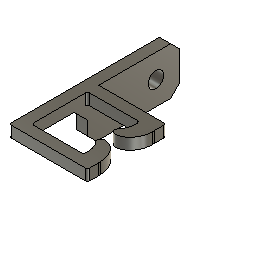
vertical (Autodesk Fusion 360 design; units mm, degrees)
Autodesk Fusion 360 part; units mm, degrees
sketch "rail-profile" plane through (0, 0, 0) normal (0, 1, 0) x (1, 0, 0)
  line L0 (-13.3, -34.5) -> (-13.3, -17.775)
  line L1 (-11.8, -16.275) -> (-1.5, -16.275)
  line L2 (0, -14.775) -> (0, 0)
  line L3 (0, 0) -> (5, 0) construction
  arc A0 (-11.8, -16.275) -> (-13.3, -17.775) centre (-11.8, -17.775) ccw
  arc A1 (-1.5, -16.275) -> (0, -14.775) centre (-1.5, -14.775) ccw
  line L4 (-12, -34.5) -> (-12, -17.775)
  arc A2 (-11.8, -17.575) -> (-12, -17.775) centre (-11.8, -17.775) ccw
  line L5 (-11.8, -17.575) -> (-1.5, -17.575)
  arc A3 (-1.5, -17.575) -> (1.3, -14.775) centre (-1.5, -14.775) ccw
  line L6 (1.3, -14.775) -> (1.3, 0)
  line L7 (-13.3, -34.5) -> (-12, -34.5)
  line L8 (0, 14.775) -> (0, 0)
  arc A4 (0, 14.775) -> (-1.5, 16.275) centre (-1.5, 14.775) ccw
  line L9 (-11.8, 16.275) -> (-1.5, 16.275)
  arc A5 (-13.3, 17.775) -> (-11.8, 16.275) centre (-11.8, 17.775) ccw
  line L10 (-13.3, 34.5) -> (-13.3, 17.775)
  line L11 (-13.3, 34.5) -> (-12, 34.5)
  line L12 (-12, 34.5) -> (-12, 17.775)
  arc A6 (-12, 17.775) -> (-11.8, 17.575) centre (-11.8, 17.775) ccw
  line L13 (-11.8, 17.575) -> (-1.5, 17.575)
  arc A7 (1.3, 14.775) -> (-1.5, 17.575) centre (-1.5, 14.775) ccw
  line L14 (1.3, 14.775) -> (1.3, 0)
  point P0 (-13.3, -16.275)
  point P1 (0, -16.275)
  dimension "d4" = 16.275
  dimension "d5" = 13.3
  dimension "d7" = 34.5
  dimension "d8" = 1.5
  dimension "d9" = 1.5
  dimension "d10" = 1.3
  constraint vertical L0
  constraint perpendicular L0 L1
  constraint perpendicular L1 L2
  constraint coincident L2.end L3.start
  constraint perpendicular L2 L3
  constraint coincident P0 L0
  constraint coincident P0 L1
  constraint tangent L0 A0
  constraint tangent L1 A0
  constraint coincident P1 L1
  constraint coincident P1 L2
  constraint tangent L1 A1
  constraint tangent L2 A1
  constraint symmetric L0.start L3 L10.start
  constraint symmetric L2.end L3 L8.end
  constraint symmetric L3 L0.end A5.start
  constraint symmetric L3 L1.start L9.start
  constraint symmetric L3 A0 A5
  constraint symmetric L3 L1.end A4.end
  constraint symmetric L3 L2.start L8.start
  constraint symmetric L3 A1 A4
  constraint symmetric L3 L4.start L11.end
  constraint symmetric L3 L4.end L12.end
  constraint symmetric L3 A2.start A6.end
  constraint symmetric L3 A2 A6
  constraint symmetric L3 L5.end L13.end
  constraint symmetric L3 A3.end A7.start
  constraint symmetric L3 A3 A7
  constraint symmetric L3 L6.end L14.end
  measures "d4" distance of L1 L3
  measures "d5" distance of P0 P1
  measures "d7" vertical distance of L0.start L3.end
  measures "d8" radius of A0
  measures "d9" radius of A1
extrude "Extrude1" add sketch "rail-profile" along normal blind 60 makes body 1
sketch "cutoout-profile" plane through (0, 0, 0) normal (-1, 0, 0) x (0, -1, 0)
  line L0 (0, -14.775) -> (0, 14.775)
  line L1 (0, 14.775) -> (-60, 14.775)
  line L2 (-60, 14.775) -> (-60, -14.775)
  line L3 (-60, -14.775) -> (0, -14.775)
  line L4 (-50.85, 4.575) -> (-60, 4.575)
  line L5 (-60, 4.575) -> (-60, -4.575)
  line L6 (-60, -4.575) -> (-50.85, -4.575)
  line L7 (-50.85, -4.575) -> (-50.85, 4.575)
  line L8 (-50.85, 4.575) -> (-60, -4.575) construction
  line L9 (-60, 4.575) -> (-50.85, -4.575) construction
  line L10 (-60, 0) -> (0, 0) construction
  line L11 (-40, -4.575) -> (-30.85, -4.575)
  line L12 (-30.85, -4.575) -> (-30.85, 4.575)
  line L13 (-30.85, 4.575) -> (-40, 4.575)
  line L14 (-40, 4.575) -> (-40, -4.575)
  line L15 (-20, -4.575) -> (-10.85, -4.575)
  line L16 (-10.85, -4.575) -> (-10.85, 4.575)
  line L17 (-10.85, 4.575) -> (-20, 4.575)
  line L18 (-20, 4.575) -> (-20, -4.575)
  point P0 (-55.425, 0)
  dimension "d13" = 9.15
  dimension "d14" = 9.15
  dimension "d24" = 60
  dimension "d25" = 0
  constraint horizontal L4
  constraint perpendicular L4 L5
  constraint parallel L4 L6
  constraint parallel L5 L7
  constraint coincident L8 P0
  constraint coincident L9 P0
  constraint midpoint L2 L10.start
  constraint coincident L10.end origin
  constraint coincident P0 L10
  constraint coincident L5 L10.start
  measures "d13" distance of L5.end L6.end
  measures "d14" distance of L4.end L5.end
extrude "Extrude2" cut sketch "cutoout-profile" against normal up to surface (1.3 mm away) contours L2 L4 L5 L6 L7 | L11 L12 L13 L14 | L15 L16 L17 L18 bodies 1
sketch "rail-body" plane through (1.3, 0, 0) normal (1, 0, 0) x (0, 1, 0) in component "cable-component"
  line L0 (50.85, 4.575) -> (60, 4.575)
  line L1 (60, 4.575) -> (60, 14.775)
  line L2 (60, 14.775) -> (0, 14.775)
  line L3 (0, 14.775) -> (0, -14.775)
  line L4 (0, -14.775) -> (60, -14.775)
  line L5 (60, -14.775) -> (60, -4.575)
  line L6 (60, -4.575) -> (50.85, -4.575)
  line L7 (50.85, -4.575) -> (50.85, 4.575)
  line L8 (30.85, 4.575) -> (40, 4.575)
  line L9 (40, 4.575) -> (40, -4.575)
  line L10 (40, -4.575) -> (30.85, -4.575)
  line L11 (30.85, -4.575) -> (30.85, 4.575)
  line L12 (10.85, 4.575) -> (20, 4.575)
  line L13 (20, 4.575) -> (20, -4.575)
  line L14 (20, -4.575) -> (10.85, -4.575)
  line L15 (10.85, -4.575) -> (10.85, 4.575)
  circle A0 centre (15.425, 0) radius 3.5
  line L16 (10.85, 4.575) -> (20, -4.575) construction
  line L17 (20, 4.575) -> (10.85, -4.575) construction
  line L18 (30.85, 4.575) -> (40, -4.575) construction
  line L19 (40, 4.575) -> (30.85, -4.575) construction
  circle A1 centre (35.425, 0) radius 3.5
  line L20 (4.85, 10.575) -> (46, 10.575)
  line L21 (46, 10.575) -> (46, -10.575)
  line L22 (46, -10.575) -> (4.85, -10.575)
  line L23 (4.85, -10.575) -> (4.85, 10.575)
  point P0 (15.425, 0)
  point P1 (35.425, 0)
  dimension "d28" = 7
  dimension "d30" = 7
  dimension "d31" = 6
  dimension "d32" = 6
  dimension "d33" = 6
  dimension "d34" = 6
  constraint coincident L12.start L15.end
  constraint coincident L13.end L14.start
  constraint coincident L12.end L13.start
  constraint coincident L14.end L15.start
  constraint midpoint L16 P0
  constraint coincident P0 A0.centre
  constraint coincident L8.start L11.end
  constraint coincident L9.end L10.start
  constraint coincident L8.end L9.start
  constraint coincident L10.end L11.start
  constraint midpoint L18 P1
  constraint coincident P1 A1.centre
  constraint horizontal L20
  constraint vertical L21
  constraint horizontal L22
  constraint vertical L23
  measures "d28" diameter of A0
  measures "d30" diameter of A1
  measures "d31" distance of L15 L23
  measures "d32" distance of L9 L21
  measures "d33" distance of L14 L22
  measures "d34" distance of L12 L20
extrude "Extrude1'" add sketch "rail-body" along normal blind 5 separate body contours L8 L9 L10 L11 | L12 L13 L14 L15 | L20 L21 L22 L23 makes body 2 in component "cable-component"
sketch "hook-body" plane through (0, 0, 10.575) normal (0, 0, 1) x (-1, 0, 0) in component "cable-component"
  line L0 (-1.3, -46) -> (-1.3, -4.85)
  line L1 (-1.3, -4.85) -> (-6.3, -4.85)
  line L2 (-6.3, -4.85) -> (-6.3, -46)
  line L3 (-6.3, -46) -> (-1.3, -46)
  line L4 (-6.3, -18.925) -> (-6.3, -11.925)
  line L5 (-6.3, -38.925) -> (-6.3, -31.925)
  line L6 (-1.3, -4.85) -> (-1.3, 25.15)
  line L7 (-1.3, 25.15) -> (-36.3, 25.15)
  line L8 (-36.3, 25.15) -> (-36.3, 20.15)
  line L9 (-36.3, 20.15) -> (-6.3, 20.15)
  line L10 (-1.3, -9.85) -> (-36.3, -9.85)
  line L11 (-1.3, -4.85) -> (-36.2454, -4.85)
  line L12 (-6.3, 20.15) -> (-6.3, -4.85)
  line L13 (-1.3, -4.85) -> (-1.3, -9.85)
  line L14 (-36.2454, -4.85) -> (-36.3, -9.85)
  dimension "d73" = 35
  dimension "d82" = 5
  dimension "d84" = 5
  dimension "d86" = 35
  constraint coincident L0.end L1.start
  constraint perpendicular L1 L6
  constraint perpendicular L6 L7
  constraint perpendicular L7 L8
  constraint coincident L0 L10.start
  constraint perpendicular L0 L10
  constraint horizontal L11
  constraint coincident L1.end L2.start
  constraint perpendicular L1 L12
  measures "d73" distance of L6 L8
  measures "d82" distance of L7 L9
  measures "d84" distance of L10 L11
  measures "d86" distance of L7 L10
extrude "Extrude3" add sketch "hook-body" against normal blind 5 contours L1 L6 L7 L8 L9 L11 L12 | L2 L10 L11 L14 bodies 2 in component "cable-component"
sketch "hook-profile" plane through (0, 0, 10.575) normal (0, 0, 1) x (-1, 0, 0) in component "cable-component"
  line L0 (-1.3, -46) -> (-1.3, 25.15)
  line L1 (-1.3, 25.15) -> (-36.3, 25.15)
  line L2 (-36.3, 25.15) -> (-36.3, 20.15)
  line L3 (-36.3, 20.15) -> (-6.3, 20.15)
  line L4 (-36.3, -9.85) -> (-6.3, -9.85)
  line L5 (-6.3, -9.85) -> (-6.3, -46)
  line L6 (-6.3, -46) -> (-1.3, -46)
  line L7 (-29.51, -3.85) -> (-36.2454, -3.85)
  spline S0 degree 5 poles (-36.2454, -3.85) (-36.2422, -3.7398) (-36.2342, -3.519) (-36.2171, -3.1868) (-36.1838, -2.7425) (-36.1211, -2.1886) (-36.0333, -1.6413) (-35.9167, -1.1062) (-35.7694, -0.588) (-35.5924, -0.09) (-35.3903, 0.3872) (-35.1691, 0.8444) (-34.935, 1.2835) (-34.692, 1.7065) (-34.4408, 2.1153) (-34.1762, 2.5107) (-33.8891, 2.8926) (-33.5692, 3.2598) (-33.2076, 3.6106) (-32.7989, 3.9423) (-32.3446, 4.252) (-31.8525, 4.536) (-31.3346, 4.7901) (-30.8054, 5.0093) (-30.2798, 5.188) (-29.7712, 5.3193) (-29.2893, 5.3956) (-28.8411, 5.4092) (-28.4314, 5.3544) (-28.0646, 5.2289) (-27.7456, 5.0354) (-27.4806, 4.7835) (-27.2769, 4.4876) (-27.1409, 4.1648) (-27.0781, 3.8331) (-27.0911, 3.5096) (-27.1789, 3.2064) (-27.3352, 2.9276) (-27.5468, 2.665) (-27.7932, 2.3973) (-28.0525, 2.1) (-28.3047, 1.7523) (-28.5366, 1.3455) (-28.7453, 0.8894) (-28.9331, 0.4032) (-29.1035, -0.0933) (-29.2575, -0.586) (-29.3866, -1.0791) (-29.4756, -1.5936) (-29.5254, -2.1319) (-29.5418, -2.6919) (-29.5361, -3.1515) (-29.5251, -3.4998) (-29.5154, -3.7331) (-29.51, -3.85) knots 0 0 0 0 0 0 0.02 0.04 0.06 0.08 0.1 0.12 0.14 0.16 0.18 0.2 0.22 0.24 0.26 0.28 0.3 0.32 0.34 0.36 0.38 0.4 0.42 0.44 0.46 0.48 0.5 0.52 0.54 0.56 0.58 0.6 0.62 0.64 0.66 0.68 0.7 0.72 0.74 0.76 0.78 0.8 0.82 0.84 0.86 0.88 0.9 0.92 0.94 0.96 0.98 1 1 1 1 1 1
  line L8 (-36.3068, -5.9745) -> (-36.184, -1.7255)
  line L9 (-28.7421, 1.2922) -> (-29.8225, -2.6884)
  line L10 (-29.6154, -1.588) -> (-29.4045, -6.112)
  line L11 (-6.3, 20.15) -> (-6.3, -4.85)
  line L12 (-6.3, -4.85) -> (-36.2454, -4.85)
  line L13 (-36.2454, -4.85) -> (-36.3, -9.85)
  line L14 (-36.2454, -4.85) -> (-36.2454, -3.85)
  line L15 (-6.3, 7.65) -> (-36.3271, 7.6919) construction
  line L16 (-29.51, -3.85) -> (-29.51, -4.85)
  spline S1 degree 5 poles (-36.2132, 19.2335) (-36.2103, 19.1233) (-36.2029, 18.9025) (-36.1868, 18.5703) (-36.1547, 18.1258) (-36.0936, 17.5717) (-36.0072, 17.0242) (-35.8922, 16.4888) (-35.7463, 15.9702) (-35.5707, 15.4717) (-35.3699, 14.9939) (-35.15, 14.5361) (-34.9171, 14.0964) (-34.6753, 13.6727) (-34.4253, 13.2632) (-34.1618, 12.867) (-33.8758, 12.4843) (-33.5569, 12.1162) (-33.1962, 11.7645) (-32.7885, 11.4316) (-32.335, 11.1207) (-31.8437, 10.8353) (-31.3265, 10.5798) (-30.798, 10.359) (-30.2729, 10.1789) (-29.7646, 10.0462) (-29.2829, 9.9685) (-28.8347, 9.9537) (-28.4249, 10.0073) (-28.0578, 10.1318) (-27.7382, 10.3244) (-27.4726, 10.5755) (-27.268, 10.8709) (-27.1311, 11.1933) (-27.0673, 11.5248) (-27.0794, 11.8484) (-27.1664, 12.1519) (-27.322, 12.431) (-27.5328, 12.6942) (-27.7785, 12.9626) (-28.0369, 13.2606) (-28.2882, 13.6091) (-28.519, 14.0165) (-28.7263, 14.4732) (-28.9128, 14.9599) (-29.0818, 15.4569) (-29.2344, 15.95) (-29.3622, 16.4434) (-29.4497, 16.9582) (-29.4981, 17.4966) (-29.5129, 18.0567) (-29.5059, 18.5163) (-29.4939, 18.8646) (-29.4836, 19.0978) (-29.4778, 19.2147) knots 0 0 0 0 0 0 0.02 0.04 0.06 0.08 0.1 0.12 0.14 0.16 0.18 0.2 0.22 0.24 0.26 0.28 0.3 0.32 0.34 0.36 0.38 0.4 0.42 0.44 0.46 0.48 0.5 0.52 0.54 0.56 0.58 0.6 0.62 0.64 0.66 0.68 0.7 0.72 0.74 0.76 0.78 0.8 0.82 0.84 0.86 0.88 0.9 0.92 0.94 0.96 0.98 1 1 1 1 1 1
  line L17 (-36.2687, 21.3582) -> (-36.1577, 17.1088)
  line L18 (-28.7243, 14.0703) -> (-29.7936, 18.054)
  line L19 (-29.5896, 16.953) -> (-29.366, 21.4764)
  line L20 (-29.4778, 19.2147) -> (-29.475, 20.2147)
  line L21 (-36.2104, 20.2335) -> (-36.2132, 19.2335)
  point P0 (-36.3271, 7.6919)
  point P1 (-27.2909, 3.0236)
  point P2 (-34.6419, 1.7831)
  point P3 (-28.2703, 1.7831)
  point P4 (-33.0367, 3.7418)
  point P5 (-35.7948, -0.6981)
  point P6 (-27.1603, 4.1663)
  point P7 (-30.1638, 5.2109)
  point P8 (-28.0744, 5.2109)
  point P9 (-29.2823, -0.6981)
  point P10 (-35.7714, 16.0803)
  point P11 (-34.6255, 13.596)
  point P12 (-33.0257, 11.6327)
  point P13 (-30.1569, 10.1556)
  point P14 (-28.0675, 10.1498)
  point P15 (-27.1505, 11.1919)
  point P16 (-27.2779, 12.3349)
  point P17 (-28.2538, 13.5782)
  point P18 (-29.2589, 16.0622)
  dimension "d92" = 1
  constraint coincident L7.start S0.end
  constraint midpoint L7.end L8
  constraint midpoint P9 L9
  constraint midpoint L7.start L10
  constraint horizontal L7
  constraint coincident L12.end L13.start
  constraint perpendicular L12 L14
  constraint midpoint L11 L15.start
  constraint coincident P0 L15.end
  constraint coincident L12 L16.end
  constraint perpendicular L12 L16
  constraint symmetric P1 L15 P16
  constraint symmetric P2 L15 P11
  constraint symmetric P3 L15 P17
  constraint symmetric P4 L15 P12
  constraint symmetric P5 L15 P10
  constraint symmetric P6 L15 P15
  constraint symmetric P7 L15 P13
  constraint symmetric P8 L15 P14
  constraint symmetric P9 L15 P18
  constraint symmetric L7.start L15 S1.end
  constraint symmetric L7.end L15 S1.start
  constraint symmetric L8.start L15 L17.start
  constraint symmetric L8.end L15 L17.end
  constraint symmetric L9.start L15 L18.start
  constraint symmetric L9.end L15 L18.end
  constraint symmetric L10.start L15 L19.start
  constraint symmetric L10.end L15 L19.end
  constraint symmetric L12.end L15 L21.start
  constraint symmetric L15 L16.end L20.end
  measures "d92" distance of L12.end L7.end
extrude "Extrude4" add sketch "hook-profile" against normal up to surface (5 mm away) contours L7 L12 L14 L16 | L3 S1 L18 L19 L20 L21 | L7 S0 L9 L10 | S1 L18 L19 | S0 L9 L10 bodies 2 in component "cable-component"
chamfer "Chamfer3" distance 6 angle 45 1 edges at (3.8, 4.85, 5.575) on bodies 2 in component "cable-component"
chamfer "Chamfer4" distance 4 angle 45 3 edges at (3.8, 46, 10.575) (3.8, 46, -10.575) (3.8, 4.85, -10.575) on bodies 2 in component "cable-component"
fillet "Fillet1" radius 1 7 edges at (36.3, 9.85, 8.075) (36.3, -25.15, 8.075) (1.3, -25.15, 8.075) (29.51, 4.85, 8.075) (29.4752, -20.15, 8.075) (6.3, -20.15, 8.075) (6.3, 4.85, 8.075) on bodies 2 in component "cable-component"
component "cable-component" placed x (1, 0, 0) y (0, 1, 0) z (0, 0, 1) at (0, 0, 0)
equation "d4 = ( 32.55 / 2 ) * 1 mm"
equation "d7 = ( 69 / 2 ) * 1 mm"
equation "d30 = d28"
equation "d32 = d31"
equation "d34 = d33"
equation "d40 = ( 5 / 2 ) * 1 mm"
equation "d72 = 35 mm"
equation "d73 = d72"
